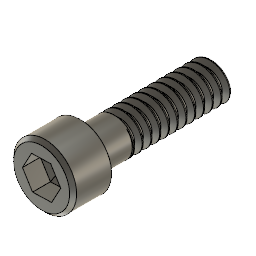
MS16995H-10-exact (Autodesk Fusion 360 design; units mm, degrees)
Autodesk Fusion 360 part; units mm, degrees
sketch "Sketch1" plane through (0, 0, 0) normal (0, 1, 0) x (1, 0, 0) in component "MS16995H-10"
  circle A0 centre (0, 0) radius 2.286
  circle A1 centre (0, 0) radius 1.397
  line L0 (-0.6574, 1.22) -> (-1.3852, 0.0406)
  line L1 (-1.3852, 0.0406) -> (-0.7278, -1.1793)
  line L2 (-0.7278, -1.1793) -> (0.6574, -1.22)
  line L3 (0.6574, -1.22) -> (1.3852, -0.0406)
  line L4 (1.3852, -0.0406) -> (0.7278, 1.1793)
  line L5 (0.7278, 1.1793) -> (-0.6574, 1.22)
  dimension "d1" = 4.572
  dimension "d2" = 2.794
  dimension "d3" = 1.2001
  constraint coincident A0.centre A1.centre
  measures "d1" diameter of A0
  measures "d2" diameter of A1
  measures "d3" distance of A0.centre L5
extrude "Extrude1" add sketch "Sketch1" along normal blind 2.794 contours A0 | A1 | L0 L1 L2 L3 L4 L5 in component "MS16995H-10"
extrude "Extrude2" add sketch "Sketch1" along normal blind 12.319 contours A1 | L0 L1 L2 L3 L4 L5 in component "MS16995H-10"
extrude "Extrude3" cut sketch "Sketch1" along normal blind 1.2954 contours L0 L1 L2 L3 L4 L5 in component "MS16995H-10"
extrude "Extrude4" cut sketch "Sketch1" along normal blind 0.508 draft -70 from surface at 1.2954 contours L0 L1 L2 L3 L4 L5 in component "MS16995H-10"
thread "Thread1" "ANSI Unified Screw Threads 0.112(#4) 4-40 UNC 3A" major diameter 2.7813 minor diameter 2.0879 pitch 0.635 angle 60 modelled right hand crest width 0.0794 on face at (1.3901, 5.969, -0.1391) from (0, 5.1752, 0) to (0, 12.319, 0) crest through (1.3906, 2.7543, 0) in component "MS16995H-10"
chamfer "Chamfer1" distance 0.254 angle 45 1 edges at (-2.1313, 0, 0.8267) in component "MS16995H-10"
fillet "Fillet1" radius 0.2032 1 edges at (-1.2965, 2.794, -0.5029) in component "MS16995H-10"
component "MS16995H-10" placed x (1, 0, 0) y (0, 1, 0) z (0, 0, 1) at (0, 0, 0)
equation "d3 = ( 0.0945 / 2 ) * 1 in"
equation "d6 = 0.11 in + 0.375 in"
equation "d11 = 0.375 * 0.75 in"
